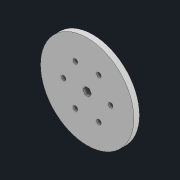
# Autodesk Inventor part: Input _Ring
Saved by Autodesk Inventor 2022 (Build 260153000, 153)
## iProperties
Created: 2022-01-11
Part Number: Input _Ring
Material: Generic
Document SubType Name: Modeling
Designer: divid
Density: 1 g/cm^3
Appearance: Default
Author: divid
Autodesk Inventor part; units mm, degrees
ref_plane "YZ Plane" through (0, 0, 0) normal (1, 0, 0) x (0, 1, 0)
ref_plane "XZ Plane" through (0, 0, 0) normal (0, 1, 0) x (-1, 0, 0)
ref_plane "XY Plane" through (0, 0, 0) normal (0, 0, 1) x (1, 0, 0)
sketch "Sketch1" plane through (0, 0, 0) normal (0, 0, 1) x (1, 0, 0)
  circle A0 centre (0, 0) radius 31.75
  dimension "d0" = 63.5
  constraints: 1 centre point, 1 coincident
  measures "d0" diameter of A0
extrude "Extrusion1" add sketch "Sketch1" along normal blind 3.81
sketch "Sketch2" plane through (0, 0, 3.81) normal (0, 0, 1) x (1, 0, 0)
  line L0 (-16, 0) -> (-8, 13.8564)
  line L1 (-8, 13.8564) -> (8, 13.8564)
  circle A0 centre (-8, 13.8564) radius 1.55
  line L2 (8, 13.8564) -> (16, 0)
  circle A1 centre (8, 13.8564) radius 1.55
  line L3 (16, 0) -> (8, -13.8564)
  circle A2 centre (16, 0) radius 1.55
  line L4 (8, -13.8564) -> (-8, -13.8564)
  circle A3 centre (8, -13.8564) radius 1.55
  line L5 (-8, -13.8564) -> (-16, 0)
  circle A4 centre (-8, -13.8564) radius 1.55
  line L6 (-16, 0) -> (-8, 13.8564)
  circle A5 centre (-16, 0) radius 1.55
  point P0 (0, 0)
  point P1 (0, 0)
  point P2 (0, 0)
  point P3 (0, 0)
  point P4 (0, 0)
  point P5 (0, 0)
  point P6 (0, 0)
  point P7 (0, 0)
  point P8 (0, 0)
  point P9 (0, 0)
  point P10 (0, 0)
  point P11 (0, 0)
  dimension "d3" = 16
  dimension "d4" = 3.1
  dimension "d7" = 360
  constraints: 14 coincident, 14 end point, 6 centre point, 45 other
  measures "d3" distance of L0.end L1.end
  measures "d4" diameter of A0
extrude "Extrusion2" cut sketch "Sketch2" against normal blind 3.81 contours L5 A5 L0 | L0 A5 L5 | A0 L1 L0 | L0 L1 A0 | A4 L4 L5 | L5 L4 A4 | A1 L2 L1 | L1 L2 A1 | A3 L3 L4 | L4 L3 A3 | A2 L3 L2 | L2 L3 A2
sketch "Sketch3" plane through (0, 0, 3.81) normal (0, 0, 1) x (1, 0, 0)
  circle A0 centre (0, 0) radius 31.75 projected
  line L0 (-2.8868, 0) -> (-1.4434, 2.5)
  line L1 (-1.4434, 2.5) -> (1.4434, 2.5)
  line L2 (1.4434, 2.5) -> (2.8868, 0)
  line L3 (2.8868, 0) -> (1.4434, -2.5)
  line L4 (1.4434, -2.5) -> (-1.4434, -2.5)
  line L5 (-1.4434, -2.5) -> (-2.8868, 0)
  dimension "d14" = 5
  constraints: 12 end point, 1 coincident, 13 other
  measures "d14" distance between parallel lines of L4 L1
extrude "Extrusion3" cut sketch "Sketch3" against normal blind 3.81 contours L0 L1 L2 L3 L4 L5
body "Solid1"
